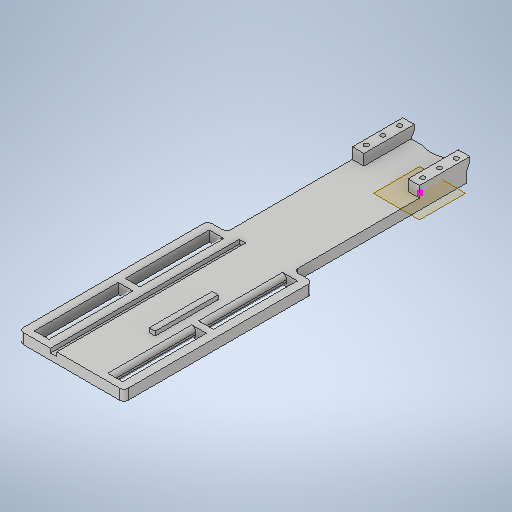
# Autodesk Inventor part: arm1_1
Saved by Autodesk Inventor 2025.1 (Build 291241000, 241)
## iProperties
Created: 2018-10-22
Part Number: arm1_1
Material: 일반
Document SubType Name: Modeling
Designer: otm09
Density: 1 g/cm^3
Appearance: 기본값
Author: otm09
Autodesk Inventor part; units mm, degrees
note: some values were not read from the file. Chosen so that the rebuilt part matches the saved one: sketch regions of "돌출1".
ref_plane "YZ Plane" through (0, 0, 0) normal (1, 0, 0) x (0, 1, 0)
ref_plane "XZ Plane" through (0, 0, 0) normal (0, 1, 0) x (-1, 0, 0)
ref_plane "XY Plane" through (0, 0, 0) normal (0, 0, 1) x (1, 0, 0)
sketch "스케치1" plane through (0, 0, 0) normal (0, 1, 0) x (-1, 0, 0)
  line L0 (0, 0) -> (32, 0)
  line L1 (32, 0) -> (32, -24)
  line L2 (32, -24) -> (0, -24)
  line L3 (0, -24) -> (0, 0)
  circle A0 centre (2.5, -4) radius 1.1
  circle A1 centre (2.5, -12) radius 1.1
  circle A2 centre (2.5, -20) radius 1.1
  circle A3 centre (29.5, -4) radius 1.1
  circle A4 centre (29.5, -12) radius 1.1
  circle A5 centre (29.5, -20) radius 1.1
  line L4 (5.5, 0) -> (26.5, 0)
  line L5 (26.5, 0) -> (26.5, -24)
  line L6 (26.5, -24) -> (5.5, -24)
  line L7 (5.5, -24) -> (5.5, 0)
  line L8 (32, 0) -> (0, 0)
  line L9 (0, 0) -> (0, 150)
  line L10 (0, 150) -> (32, 150)
  line L11 (32, 150) -> (32, 0)
  line L12 (41, 150) -> (-9, 150)
  line L13 (-9, 150) -> (-9, 60)
  line L14 (-9, 60) -> (41, 60)
  line L15 (41, 60) -> (41, 150)
  line L16 (32, 63.3333) -> (37, 63.3333)
  line L17 (37, 63.3333) -> (37, 103.3333)
  line L18 (37, 103.3333) -> (32, 103.3333)
  line L19 (32, 103.3333) -> (32, 63.3333)
  line L20 (32, 106.6667) -> (37, 106.6667)
  line L21 (37, 106.6667) -> (37, 146.6667)
  line L22 (37, 146.6667) -> (32, 146.6667)
  line L23 (32, 146.6667) -> (32, 106.6667)
  line L24 (0, 63.3333) -> (-5, 63.3333)
  line L25 (-5, 63.3333) -> (-5, 103.3333)
  line L26 (-5, 103.3333) -> (0, 103.3333)
  line L27 (0, 103.3333) -> (0, 63.3333)
  line L28 (0, 106.6667) -> (-5, 106.6667)
  line L29 (-5, 106.6667) -> (-5, 146.6667)
  line L30 (-5, 146.6667) -> (0, 146.6667)
  line L31 (0, 146.6667) -> (0, 106.6667)
  dimension "d0" = 32
  dimension "d1" = 24
  dimension "d2" = 2.2
  dimension "d3" = 4
  dimension "d6" = 8
  dimension "d11" = 2.5
  dimension "d12" = 2.2
  dimension "d15" = 8
  dimension "d20" = 4
  dimension "d21" = 2.5
  dimension "d22" = 21
  dimension "d23" = 5.5
  dimension "d28" = 150
  dimension "d29" = 50
  dimension "d30" = 90
  dimension "d31" = 9
  dimension "d32" = 5
  dimension "d33" = 40
  dimension "d34" = 40
  dimension "d35" = 3.3333
  dimension "d36" = 3.3333
  dimension "d37" = 5
  dimension "d38" = 5
  dimension "d45" = 3.3333
  dimension "d46" = 40
  dimension "d47" = 3.3333
  dimension "d48" = 40
  constraints: 64 end point, 16 parallel, 8 horizontal, 8 perpendicular, 8 point on line, 6 centre point, 2 vertical, 8 other
  measures "d0" distance of L1.end L2.end
  measures "d1" distance of L0.end L1.end
  measures "d2" diameter of A0
  measures "d3" distance from line of A0.centre L0
  measures "d6" distance of A0.centre A1.centre
  measures "d11" distance from line of L3 A0.centre
  measures "d12" diameter of A3
  measures "d15" distance of A3.centre A4.centre
  measures "d20" distance from line of A3.centre L0
  measures "d21" distance from line of A3.centre L1
  measures "d22" distance between parallel lines of L5 L7
  measures "d23" distance between parallel lines of L3 L7
  measures "d28" distance of L8.end L9.end
  measures "d29" distance of L14.end L13.end
  measures "d30" distance of L13.end L12.end
  measures "d31" distance between parallel lines of L15 L11
  measures "d32" distance of L18.end L17.end
  measures "d33" distance of L17.end L16.end
  measures "d34" distance of L21.end L20.end
  measures "d35" distance between parallel lines of L16 L14
  measures "d36" distance between parallel lines of L20 L18
  measures "d37" distance of L25.end L26.end
  measures "d38" distance of L29.end L30.end
  measures "d45" distance between parallel lines of L24 L14
  measures "d46" distance of L24.end L25.end
  measures "d47" distance between parallel lines of L28 L26
  measures "d48" distance of L28.end L29.end
extrude "돌출1" add sketch "스케치1" along normal blind 5.2 contours L0 L7 L2 L3 | L0 L1 L2 L5
extrude "돌출2" add sketch "스케치1" against normal blind 5 contours L9 L14 L11 L0 | L0 L7 L2 L3 | L0 L5 L2 L7 | L14 L13 L12 L9 L30 L29 L28 L26 L25 L24 | L9 L10 L11 L14 | L0 L1 L2 L5 | L11 L16 L17 L18 L20 L21 L22 L12 L15 L14
fillet "모깎기1" radius 2 14 edges at (0, 0, 83.3333) (0, 0, 126.6667) (-32, 0, 126.6667) (-32, 0, 83.3333) (0, -5, 83.3333) (-32, -5, 83.3333) (0, -5, 126.6667) (-32, -5, 126.6667) (9, -2.5, 150) (-41, -2.5, 150) (9, -2.5, 60) (-41, -2.5, 60) (-32, -2.5, 60) (0, -2.5, 60)
sketch "스케치2" plane through (0, -5, 0) normal (0, -1, 0) x (1, 0, 0)
  circle A0 centre (-16, -34.5) radius 13
  circle A1 centre (-29.5, -20) radius 1.1 projected
  line L0 (0, -24) -> (0, 58) projected
  line L1 (0, 0) -> (0, -24) projected
  line L2 (-26.5, -24) -> (-32, -24) projected
  line L3 (0, -22.5) -> (-32, -22.5)
  line L4 (-32, -22.5) -> (-32, -24)
  line L5 (-32, -24) -> (0, -24)
  line L6 (0, -24) -> (0, -22.5)
  line L7 (-32, -24) -> (0, -24) projected
  dimension "d40" = 26
  dimension "d41" = 14.5
  dimension "d42" = 16
  dimension "d57" = 1.5
  constraints: 8 end point, 2 parallel, 1 centre point, 1 collinear, 1 horizontal, 1 perpendicular, 1 point on line
  measures "d40" diameter of A0
  measures "d41" vertical distance of A1.centre A0.centre
  measures "d42" distance from line of A0.centre L0
  measures "d57" distance between parallel lines of L2 L3
extrude "돌출3" cut sketch "스케치2" against normal blind 5 contours A0 L5 | L5 A0 L3 | A0 L3 L0 L5 | L5 L2 L4 L3 A0 | L3 A0
sketch "스케치3" plane through (0, -5, 0) normal (0, -1, 0) x (1, 0, 0)
  circle A0 centre (-2.5, -4) radius 1.1 projected
  circle A1 centre (-2.5, -4) radius 2.1
  circle A2 centre (-2.5, -12) radius 1.1 projected
  circle A3 centre (-2.5, -12) radius 2.1
  circle A4 centre (-2.5, -20) radius 1.1 projected
  circle A5 centre (-2.5, -20) radius 2.1
  circle A6 centre (-29.5, -4) radius 1.1 projected
  circle A7 centre (-29.5, -4) radius 2.1
  circle A8 centre (-29.5, -12) radius 1.1 projected
  circle A9 centre (-29.5, -12) radius 2.1
  circle A10 centre (-29.5, -20) radius 1.1 projected
  circle A11 centre (-29.5, -20) radius 2.1
  point P0 (0, 0)
  dimension "d49" = 4.2
  dimension "d50" = 4.2
  dimension "d51" = 4.2
  dimension "d52" = 4.2
  dimension "d53" = 4.2
  dimension "d54" = 4.2
  constraints: 6 centre point, 6 coincident
  measures "d49" diameter of A1
  measures "d50" diameter of A3
  measures "d51" diameter of A5
  measures "d52" diameter of A7
  measures "d53" diameter of A9
  measures "d54" diameter of A11
extrude "돌출4" cut sketch "스케치3" against normal blind 8.2
chamfer "모따기1" distance 3 distance2 1.5 1 edges at (-29.25, 0, -24) measured on face at (-28.3333, 3.4667, -24)
chamfer "모따기2" distance 3 distance2 1.5 1 edges at (-2.75, 0, -24) measured on face at (-1.8333, 1.7333, -24)
sketch "스케치4" plane through (0, 0, 0) normal (0, 1, 0) x (1, 0, 0)
  line L0 (-39, -150) -> (7, -150) projected
  line L1 (0, -150) -> (-9, -150)
  line L2 (-9, -150) -> (-32, -150)
  line L3 (-9, -150) -> (-6, -150)
  line L4 (-32, -150) -> (-23, -150)
  line L5 (-23, -150) -> (-26, -150)
  line L6 (-26, -150) -> (-26, -30)
  line L7 (-26, -150) -> (-23, -150)
  line L8 (-23, -150) -> (-23, -30)
  line L9 (-23, -30) -> (-26, -30)
  line L10 (-26, -30) -> (-26, -150)
  line L11 (-9, -150) -> (-6, -150)
  line L12 (-6, -150) -> (-6, -90)
  line L13 (-6, -90) -> (-9, -90)
  line L14 (-9, -90) -> (-9, -150)
  line L15 (-26, -60) -> (-23, -60)
  point P0 (0, 0)
  dimension "d64" = 9
  dimension "d65" = 23
  dimension "d66" = 3
  dimension "d68" = 9
  dimension "d69" = 3
  dimension "d70" = 120
  dimension "d71" = 60
  constraints: 30 end point, 8 point on line, 4 parallel, 4 perpendicular, 2 horizontal
  measures "d64" distance of L1.start L1.end
  measures "d65" distance of L1.end L2.end
  measures "d66" distance of L1.end L3.end
  measures "d68" distance of L2.end L4.end
  measures "d69" distance of L4.end L5.end
  measures "d70" distance of L5.end L6.end
  measures "d71" distance of L12.end L11.end
extrude "돌출5" cut sketch "스케치4" against normal blind 2 contours L6 L15 L8 L0
ref_plane "작업 평면1" through (0, 2, 0) normal (0, 1, 0) x (1, 0, 0)
sketch "스케치6" plane through (0, 2, 0) normal (0, 1, 0) x (1, 0, 0)
  point P0 (0, 0)
sketch "스케치7" plane through (0, 0, 0) normal (0, 1, 0) x (1, 0, 0)
  line L0 (7, -150) -> (-39, -150) projected
  line L1 (0, -150) -> (-6.1, -150)
  line L2 (-6.1, -150) -> (-8.9, -150)
  line L3 (-8.9, -150) -> (-8.9, -90)
  line L4 (-8.9, -90) -> (-6.1, -90)
  line L5 (-6.1, -90) -> (-6.1, -150)
  line L6 (-6.1, -90) -> (-8.9, -90)
  line L7 (-8.9, -90) -> (-8.9, -120)
  line L8 (-8.9, -120) -> (-6.1, -120)
  line L9 (-6.1, -120) -> (-6.1, -90)
  point P0 (0, 0)
  dimension "d79" = 6.1
  dimension "d80" = 2.8
  dimension "d81" = 60
  constraints: 18 end point, 4 parallel, 2 horizontal, 2 perpendicular, 2 point on line, 1 midpoint
  measures "d79" distance of L1.start L1.end
  measures "d80" distance of L3.end L4.end
  measures "d81" distance of L2.end L3.end
extrude "돌출7" add sketch "스케치7" along normal blind 2 contours L8 L3 L4 L5
equation "\"d23\" = -0.5 * d22 + 0.5 * d0"
equation "\"d35\" = -0.333333 * d34 + 0.333333 * d30 - 0.333333 * d33"
equation "\"d36\" = -0.333333 * d34 + 0.333333 * d30 - 0.333333 * d33"
equation "\"d45\" = -0.333333 * d34 + 0.333333 * d30 - 0.333333 * d33"
equation "\"d47\" = -0.333333 * d34 + 0.333333 * d30 - 0.333333 * d33"
